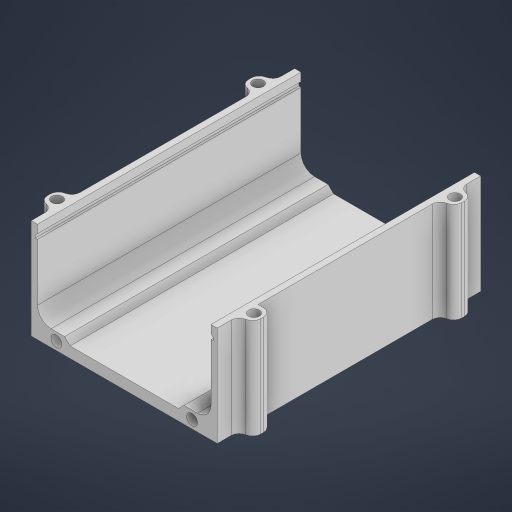
# Autodesk Inventor part: Discovery boar holder
Saved by Autodesk Inventor 2023 (Build 270158000, 158)
## iProperties
Created: 2024-01-04
Part Number: Discovery boar holder
Material: Generic
Document SubType Name: Modeling
Designer: nick_
Density: 1 g/cm^3
Appearance: Default
Author: nick_
Autodesk Inventor part; units mm, degrees
ref_plane "YZ Plane" through (0, 0, 0) normal (1, 0, 0) x (0, 1, 0)
ref_plane "XZ Plane" through (0, 0, 0) normal (0, 1, 0) x (-1, 0, 0)
ref_plane "XY Plane" through (0, 0, 0) normal (0, 0, 1) x (1, 0, 0)
sketch "Sketch1" plane through (0, 0, 0) normal (0, 0, 1) x (1, 0, 0)
  line L0 (0, 0) -> (-34.25, 0)
  line L1 (-34.25, 0) -> (-34.25, 36.8)
  line L2 (-34.25, 36.8) -> (-31.95, 36.8)
  line L3 (-31.95, 36.8) -> (-31.95, 33.8)
  line L4 (-31.95, 33.8) -> (-32.75, 33.8)
  line L5 (-32.75, 33.8) -> (-32.75, 32)
  line L6 (-32.75, 32) -> (-31.95, 32)
  line L7 (-31.95, 32) -> (-31.95, 6)
  line L8 (-31.95, 6) -> (0, 6)
  line L9 (0, 6) -> (0, 0)
  point P0 (-32.75, 32.9)
  point P1 (0, 3)
  dimension "d0" = 6
  dimension "d2" = 0.8
  dimension "d3" = 3
  dimension "d4" = 1.8
  dimension "d5" = 1.5
  dimension "d9" = 26
  dimension "d15" = 65.5
  constraints: 20 end point, 7 perpendicular, 2 midpoint, 1 horizontal, 1 parallel, 1 point on line, 1 vertical
  measures "d0" distance between parallel lines of L0 L8
  measures "d2" distance between parallel lines of L3 L5
  measures "d3" distance of L2.end L3.end
  measures "d4" distance of L4.end L5.end
  measures "d5" distance between parallel lines of L1 L5
  measures "d9" distance of L6.end L7.end
  measures "d15" diameter of L5 L9
extrude "Extrusion1" add sketch "Sketch1" along normal blind 97
sketch "Sketch5" plane through (-34.25, 36.8, 0) normal (0, 1, 0) x (1, 0, 0)
  line L0 (0, 0) -> (0, -97) projected
  line L1 (0, -8) -> (-5, -8)
  line L2 (-5, -8) -> (-5, -15)
  line L3 (-5, -15) -> (0, -15)
  line L4 (0, -15) -> (0, -8)
  line L5 (0, -89) -> (-5, -89)
  line L6 (-5, -89) -> (-5, -82)
  line L7 (-5, -82) -> (0, -82)
  line L8 (0, -82) -> (0, -89)
  line L9 (2.3, -97) -> (0, -97) projected
  point P0 (34.25, 0)
  point P1 (1.15, -97)
  point P2 (0, -82)
  point P3 (0, -15)
  dimension "d23" = 5
  dimension "d24" = 7
  dimension "d25" = 8
  dimension "d26" = 5
  dimension "d27" = 7
  dimension "d28" = 8
  constraints: 16 end point, 4 parallel, 2 horizontal, 2 perpendicular, 2 point on line, 1 midpoint
  measures "d23" distance of L3.end L2.end
  measures "d24" distance of L2.end L1.end
  measures "d25" distance from line of L0.start L1
  measures "d26" distance of L6.end L7.end
  measures "d27" distance of L5.end L6.end
  measures "d28" distance from line of point (1.15, -97) L5
extrude "Extrusion3" add sketch "Sketch5" against normal up to surface (36.8 mm away)
fillet "Fillet2" radius 3 4 edges at (-39.25, 18.4, 15) (-39.25, 18.4, 8) (-39.25, 18.4, 89) (-39.25, 18.4, 82)
sketch "Sketch6" plane through (-34.25, 36.8, 0) normal (0, 1, 0) x (1, 0, 0)
  arc A0 (-2, -82) -> (-5, -85) centre (-2, -85) ccw construction
  line L0 (-5, -85) -> (-5, -86) construction
  arc A1 (-5, -86) -> (-2, -89) centre (-2, -86) ccw construction
  line L1 (-2, -89) -> (0, -89) construction
  line L2 (0, -89) -> (0, -97) construction
  line L3 (2.3, -97) -> (0, -97) construction
  line L4 (2.3, 0) -> (2.3, -97) construction
  line L5 (2.3, 0) -> (0, 0) construction
  line L6 (0, 0) -> (0, -8) construction
  line L7 (0, -8) -> (-2, -8) construction
  arc A2 (-2, -8) -> (-5, -11) centre (-2, -11) ccw construction
  line L8 (-5, -11) -> (-5, -12) construction
  arc A3 (-5, -12) -> (-2, -15) centre (-2, -12) ccw construction
  line L9 (-2, -15) -> (0, -15) construction
  line L10 (0, -15) -> (0, -82) construction
  line L11 (0, -82) -> (-2, -82) construction
  point P0 (34.25, 0)
  point P1 (-2, -11.5)
  point P2 (-5, -11.5)
  point P3 (-2, -85.5)
  point P4 (-5, -85.5)
  constraints: 2 horizontal alignment, 2 midpoint, 2 vertical alignment
hole "Hole1" at (-36.25, 36.8, 11.5) at (-36.25, 36.8, 85.5) direction (0, -1, 0) diameter 4 end through all
mirror "Mirror1" about plane through (0, 0, 0) normal (1, 0, 0) of "Extrusion1", "Extrusion3", "Fillet2", "Hole1"
fillet "Fillet3" radius 5 2 edges at (-31.95, 6, 48.5) (31.95, 6, 48.5)
fillet "Fillet4" radius 3 7 edges at (-34.25, 18.4, 89) (-34.25, 18.4, 82) (-34.25, 18.4, 15) (-34.25, 18.4, 8) (34.25, 18.4, 89) (34.25, 18.4, 15) (34.25, 18.4, 8)
chamfer "Chamfer2" distance 0.8 angle 45 2 edges at (-32.75, 33.8, 48.5) (32.75, 33.8, 48.5)
sketch "Sketch7" plane through (0, 0, 0) normal (0, 0, -1) x (-1, 0, 0)
  line L0 (26.95, 6) -> (-26.95, 6) projected
  line L1 (-20.95, 6) -> (20.95, 6)
  line L2 (20.95, 6) -> (20.95, 4)
  line L3 (20.95, 4) -> (-20.95, 4)
  line L4 (-20.95, 4) -> (-20.95, 6)
  point P0 (0, 0)
  point P1 (20.95, 6)
  dimension "d44" = 2
  dimension "d45" = 6
  dimension "d46" = 6
  constraints: 8 end point, 2 parallel, 1 horizontal, 1 perpendicular, 1 point on line
  measures "d44" distance of L1.end L2.end
  measures "d45" horizontal distance of L3.end L0.end
  measures "d46" horizontal distance of L0.start L2.end
extrude "Extrusion4" cut sketch "Sketch7" against normal through all
chamfer "Chamfer3" distance 1 angle 45 4 edges at (20.95, 4, 48.5) (20.95, 6, 48.5) (-20.95, 4, 48.5) (-20.95, 6, 48.5)
sketch "Sketch8" plane through (0, 0, 0) normal (0, 0, -1) x (-1, 0, 0)
  line L0 (34.25, 0) -> (-34.25, 0) projected
  point P0 (0, 0)
  point P1 (-25, 3)
  point P2 (25, 3)
  point P3 (0, 0)
  dimension "d52" = 50
  dimension "d53" = 25
  dimension "d54" = 3
  constraints: 1 horizontal alignment, 1 midpoint
  measures "d52" distance of point (25, 3) point (-25, 3)
  measures "d53" horizontal distance of point (0, 0) point (-25, 3)
  measures "d54" distance from line of L0 point (25, 3)
hole "Hole2" at (25, 3, 0) at (-25, 3, 0) direction (0, 0, 1) diameter 4 end through all
sketch "Sketch2" plane through (-31.95, 6, 97) normal (0, 1, 0) x (1, 0, 0)
  line L0 (63.9, 97) -> (0, 97) construction
  line L1 (0, 97) -> (0, 0) construction
  line L2 (0, 0) -> (63.9, 0) construction
  line L3 (63.9, 97) -> (63.9, 0) construction
  line L4 (15.3721, 48.5) -> (48.5279, 48.5) construction
  line L5 (15.3721, 46.3) -> (48.5279, 46.3)
  line L6 (48.5279, 50.7) -> (15.3721, 50.7)
  arc A0 (15.3721, 50.7) -> (15.3721, 46.3) centre (15.3721, 48.5) ccw
  arc A1 (48.5279, 46.3) -> (48.5279, 50.7) centre (48.5279, 48.5) ccw
  line L7 (66.2, 97) -> (66.2, 0) projected
  point P0 (31.95, 97)
  point P1 (31.95, 48.5)
  point P2 (31.95, 97)
  point P3 (66.2, 48.5)
  dimension "d12" = 2.2
  constraints: 8 end point, 4 point on circle, 4 tangent, 3 midpoint, 2 centre point, 2 parallel, 1 horizontal alignment, 1 vertical alignment
  measures "d12" radius of A0
equation "\"d26\" = d23"
equation "\"d27\" = d24"
equation "\"d28\" = d25"
equation "\"d46\" = d45"
equation "\"d53\" = 0.5 * d52"
body "Solid1"
